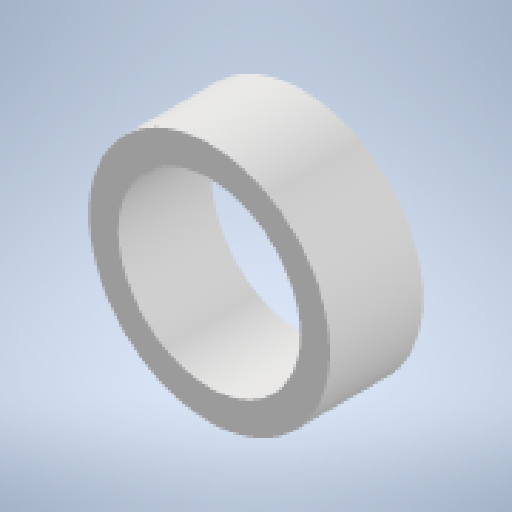
# Autodesk Inventor part: Separadores
Saved by Autodesk Inventor 2024 (Build 280153000, 153)
## iProperties
Created: 2025-03-07
Part Number: Separadores
Material: Genérico
Document SubType Name: Modeling
Designer: sergi
Density: 1 g/cm^3
Appearance: Valor por defecto
Author: sergi
Autodesk Inventor part; units mm, degrees
ref_plane "YZ Plane" through (0, 0, 0) normal (1, 0, 0) x (0, 1, 0)
ref_plane "XZ Plane" through (0, 0, 0) normal (0, 1, 0) x (-1, 0, 0)
ref_plane "XY Plane" through (0, 0, 0) normal (0, 0, 1) x (1, 0, 0)
sketch "Boceto1" plane through (0, 0, 0) normal (0, 0, 1) x (1, 0, 0)
  circle A0 centre (11, 11) radius 7.3 projected
  circle A1 centre (11, 11) radius 9.7
  circle A2 centre (11, 11) radius 7.5
  point P0 (0, 0)
  dimension "d0" = 2.4
  dimension "d3" = 0.2
  constraints: 2 centre point
  measures "d0" radial gap between concentric circles of A0 A1
  measures "d3" radial gap between concentric circles of A0 A2
extrude "Extrusión1" add sketch "Boceto1" along normal blind 8 contours A1
